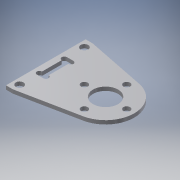
# Autodesk Inventor part: 肩_サブフレーム_1_1
Saved by Autodesk Inventor 2018 (Build 220112000, 112)
## iProperties
Category: 肩
Created: 2016-05-05
Part Number: 肩_サブフレーム_1_1
Material: アルミニウム 2014-T4
Document SubType Name: Modeling
Designer: hiroaki
Density: 2.8 g/cm^3
Appearance: サテン
Mass: 3.06212 g
Surface Area: 18.1271 cm^2
Volume: 1.09361 cm^3
Author: hiroaki
Autodesk Inventor part; units mm, degrees
ref_plane "YZ Plane" through (0, 0, 0) normal (1, 0, 0) x (0, 1, 0)
ref_plane "XZ Plane" through (0, 0, 0) normal (0, 1, 0) x (-1, 0, 0)
ref_plane "XY Plane" through (0, 0, 0) normal (0, 0, 1) x (1, 0, 0)
sketch "スケッチ1" plane through (0, 0, 0) normal (0, 0, 1) x (1, 0, 0)
  circle A0 centre (0, 0) radius 10.5 construction
  line L0 (-12, 10.583) -> (-12, -10.583) construction
  arc A1 (0, 16) -> (-12, 10.583) centre (0, 0) ccw construction
  line L1 (0, 16) -> (33.5167, 16) construction
  line L2 (33.5167, 16) -> (33.5167, -16) construction
  line L3 (33.5167, -16) -> (0, -16) construction
  arc A2 (-12, -10.583) -> (0, -16) centre (0, 0) ccw construction
  circle A3 centre (0, 8.5) radius 1.35
  circle A4 centre (-8.5, 0) radius 1.35
  circle A5 centre (0, -8.5) radius 1.35
  circle A6 centre (8.5, 0) radius 1.35
  circle A7 centre (0, 0) radius 5.05
  circle A8 centre (0, 0) radius 16 construction
  line L4 (-21.5, 6) -> (-19, 6) construction
  line L5 (-19, 6) -> (-19, -6) construction
  line L6 (-19, -6) -> (-21.5, -6) construction
  line L7 (-21.5, -6) -> (-21.5, 6) construction
  circle A9 centre (0, 0) radius 19 construction
  line L8 (-18.95, 6.05) -> (-21.55, 6.05) construction
  line L9 (-21.55, 6.05) -> (-21.55, -6.05) construction
  line L10 (-21.55, -6.05) -> (-18.95, -6.05) construction
  line L11 (-18.95, -6.05) -> (-18.95, 6.05) construction
  circle A10 centre (-21.55, 5) radius 1.05 construction
  line L12 (-18.95, 6.05) -> (-21.55, 6.05)
  arc A11 (-21.55, 6.05) -> (-21.55, 3.95) centre (-21.55, 5) ccw
  line L13 (-21.55, 3.95) -> (-21.55, -3.95)
  line L14 (-20.25, 6.05) -> (-20.25, -6.05) construction
  line L15 (-21.55, 0) -> (-19, 0) construction
  arc A12 (-21.55, -3.95) -> (-21.55, -6.05) centre (-21.55, -5) ccw
  line L16 (-21.55, -6.05) -> (-18.95, -6.05)
  line L17 (-18.95, 3.95) -> (-18.95, -3.95)
  arc A13 (-18.95, 3.95) -> (-18.95, 6.05) centre (-18.95, 5) ccw
  arc A14 (-18.95, -6.05) -> (-18.95, -3.95) centre (-18.95, -5) ccw
  line L18 (-24, 6) -> (-24, -6)
  circle A15 centre (-21.5, 13) radius 1.55
  circle A16 centre (-21.5, -13) radius 1.55
  line L19 (-24, 16) -> (-21.201, 16)
  line L20 (-24, -16) -> (-21.201, -16)
  arc A17 (2.2701, -11.2737) -> (2.2701, 11.2737) centre (0, 0) ccw
  line L21 (-24, 16) -> (-24, 6)
  circle A18 centre (-21.5, 13) radius 3 construction
  line L22 (-24, -16) -> (-24, -6)
  line L23 (-21.201, 16) -> (2.2701, 11.2737)
  line L24 (2.2701, -11.2737) -> (-21.201, -16)
  point P0 (-12, 0)
  point P1 (-20.275, 0)
  dimension "d29" = 2.1
  dimension "d0" = 21
  dimension "d1" = 16
  dimension "d2" = 12
  dimension "d3" = 8.5
  dimension "d4" = 2.7
  dimension "d7" = 360
  dimension "d9" = 10.1
  dimension "d10" = 2.5
  dimension "d11" = 3
  dimension "d27" = 10
  dimension "d30" = 0.05
  dimension "d31" = 7
  dimension "d33" = 3.1
  dimension "d41" = 2.5
  dimension "d43" = 1
  constraints: 50 end point, 18 centre point, 14 point on circle, 11 tangent, 8 coincident, 6 midpoint, 6 symmetric about line, 5 parallel, 5 perpendicular, 4 collinear, 4 horizontal, 4 vertical, 4 vertical alignment, 3 horizontal alignment, 2 equal radius, 1 point on line, 16 other
  measures "d0" diameter of A0
  measures "d1" radius of A1
  measures "d2" distance from line of point (0, 0) L0
  measures "d3" distance of point (0, 0) A3.centre
  measures "d4" diameter of A3
  measures "d9" diameter of A7
  measures "d10" distance of L4.start L4.end
  measures "d11" radial gap between concentric circles of A8 A9
  measures "d27" distance between parallel lines of L1 L4
  measures "d30" distance between parallel lines of L8 L4
  measures "d31" distance from line of L4 A15.centre
  measures "d33" diameter of A15
  measures "d41" distance between parallel lines of L18 L7
  measures "d43" radial gap between concentric circles of A17 A0
extrude "押し出し1" add sketch "スケッチ1" along normal blind 1.5
equation "\"d27\" = d21"
equation "\"d31\" = d23"
equation "\"d21\" = 10"
equation "\"d23\" = 7"
